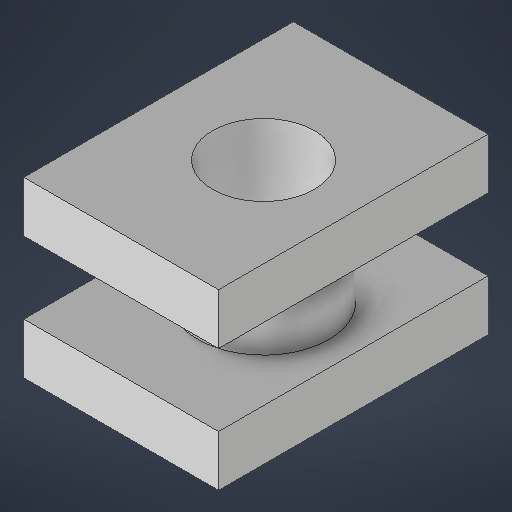
# Autodesk Inventor part: MMAE 232 CAD Assignment 2 Rubber Grommet-Nicholas Skiba
Saved by Autodesk Inventor 2026.1 (Build 301233000, 233)
## iProperties
Created: 2025-08-27
Part Number: MMAE 232 CAD Assignment 2 Rubber Grommet-Nicholas Skiba
Material: Generic
Document SubType Name: Modeling
Designer: Nick
Density: 1 g/cm^3
Appearance: Default
Author: Nick
Autodesk Inventor part; units mm, degrees
ref_plane "YZ Plane" through (0, 0, 0) normal (1, 0, 0) x (0, 1, 0)
ref_plane "XZ Plane" through (0, 0, 0) normal (0, 1, 0) x (-1, 0, 0)
ref_plane "XY Plane" through (0, 0, 0) normal (0, 0, 1) x (1, 0, 0)
sketch "Sketch1" plane through (0, 0, 0) normal (0, 1, 0) x (-1, 0, 0)
  arc A0 (1.75, 1.3) -> (1.75, -1.3) centre (0, 0) ccw
  circle A1 centre (0, 0) radius 1.7
  line L0 (0, 0) -> (0, 1.3)
  line L1 (3.5, 1.3) -> (3.5, -1.3)
  line L2 (0, 1.3) -> (1.0954, 1.3)
  line L3 (1.75, 1.3) -> (3.5, 1.3)
  line L4 (3.5, -1.3) -> (1.75, -1.3)
  dimension "d1" = 3.4
  dimension "d0" = 4.36
  dimension "d2" = 1.3
  dimension "d3" = 3.5
  dimension "d4" = 2.6
  constraints: 10 end point, 5 perpendicular, 2 coincident, 2 point on circle, 1 centre point, 1 vertical, 3 other
  measures "d0" diameter of A0
  measures "d2" distance of L0.start L0.end
  measures "d3" distance of L0.end L1.start
  measures "d4" distance of L1.start L1.end
extrude "Extrusion1" add sketch "Sketch1" along normal blind 2.4
sketch "Sketch2" plane through (0, 2.4, 0) normal (0, 1, 0) x (1, 0, 0)
  circle A0 centre (0, 0) radius 1.7
  line L0 (0, 0) -> (0, 4.5)
  line L1 (0, 4.5) -> (3, 4.5)
  line L2 (3, 4.5) -> (-3.5, 4.5)
  line L3 (-3.5, 4.5) -> (-3.5, -4.5)
  line L4 (-3.5, -4.5) -> (3, -4.5)
  line L5 (3, -4.5) -> (3, 4.5)
  dimension "d7" = 4.5
  dimension "d8" = 3
  dimension "d9" = 9
  constraints: 12 end point, 2 parallel, 2 perpendicular, 1 centre point, 1 coincident, 1 horizontal, 1 vertical
  measures "d7" distance of L0.start L0.end
  measures "d8" distance of L0.end L1.end
  measures "d9" distance of L3.end L2.end
extrude "Extrusion2" add sketch "Sketch2" along normal blind 1.7
sketch "Sketch3" plane through (0, 0, 0) normal (0, -1, 0) x (1, 0, 0)
  line L0 (-3.5, 4.5) -> (3, 4.5) projected
  line L1 (3, 4.5) -> (3, -4.5) projected
  line L2 (-3.5, 4.5) -> (3, 4.5)
  line L3 (3, 4.5) -> (3, -4.5)
  line L4 (3, -4.5) -> (-3.5, -4.5)
  line L5 (-3.5, -4.5) -> (-3.5, 4.5)
  point P0 (0, 0)
  constraints: 8 end point, 2 parallel, 1 horizontal, 1 perpendicular
extrude "Extrusion3" add sketch "Sketch3" along normal blind 1.7
sketch "Sketch4" plane through (0, 0, 0) normal (0, 1, 0) x (1, 0, 0)
  circle A0 centre (0, 0) radius 1.7
  constraints: 1 centre point, 1 coincident
extrude "Extrusion4" cut sketch "Sketch4" against normal blind 1.7
body "Solid1"
